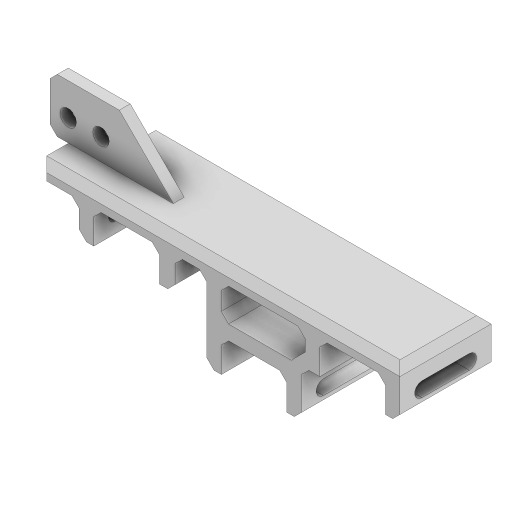
# Autodesk Inventor part: adapter_ver.1
Saved by Autodesk Inventor 2024 (Build 280153000, 153)
## iProperties
Created: 2023-11-09
Part Number: adapter_ver.1
Material: 一般
Document SubType Name: Modeling
Designer: moonshot
Density: 1 g/cm^3
Appearance: 既定
Author: moonshot
Autodesk Inventor part; units mm, degrees
ref_plane "YZ Plane" through (0, 0, 0) normal (1, 0, 0) x (0, 1, 0)
ref_plane "XZ Plane" through (0, 0, 0) normal (0, 1, 0) x (-1, 0, 0)
sketch "スケッチ1" plane through (0, 0, 0) normal (0, 0, 1) x (1, 0, 0)
  line L0 (94.5, 17.4383) -> (94.5, 4.4383)
  line L1 (67.5, 4.4383) -> (67.5, -8.5617)
  line L2 (0, -17.748) -> (0, 46.5561) projected
  line L3 (45.5, -8.5617) -> (45.5, 0.4383)
  line L4 (45.5, 0.4383) -> (63.5, 0.4383)
  line L5 (63.5, 0.4383) -> (63.5, -8.5617)
  line L6 (67.5, -8.5617) -> (63.5, -8.5617)
  line L7 (45.5, -8.5617) -> (41.5, -8.5617)
  line L8 (72.5, 4.4383) -> (72.5, 13.4383)
  line L9 (72.5, 13.4383) -> (90.5, 13.4383)
  line L10 (90.5, 13.4383) -> (90.5, 4.4383)
  line L11 (45.5, -8.5617) -> (55.5, -8.5617) construction
  line L12 (55.5, -8.5617) -> (55.5, 0.4383) construction
  line L13 (50.5, -8.5617) -> (50.5, 17.1682) construction
  line L14 (28.5, 4.4383) -> (28.5, 13.4383)
  line L15 (28.5, 13.4383) -> (10.5, 13.4383)
  line L16 (10.5, 13.4383) -> (10.5, 4.4383)
  line L17 (0, 17.4383) -> (0, 13.4383)
  line L18 (0, 17.4383) -> (94.5, 17.4383)
  line L19 (94.5, 4.4383) -> (90.5, 4.4383)
  line L20 (72.5, 4.4383) -> (67.5, 4.4383)
  line L21 (6.5, 4.4383) -> (10.5, 4.4383)
  line L22 (6.5, 4.4383) -> (6.5, 13.4383)
  line L23 (6.5, 13.4383) -> (0, 13.4383)
  line L24 (72.5, 4.4383) -> (82.5, 4.4383) construction
  line L25 (82.5, 4.4383) -> (82.5, 13.4383) construction
  line L26 (77.5, 4.4383) -> (77.5, 37.3698) construction
  line L27 (28.5, 4.4383) -> (18.5, 4.4383) construction
  line L28 (18.5, 4.4383) -> (18.5, 13.4383) construction
  line L29 (23.5, 4.4383) -> (23.5, 33.4166) construction
  line L30 (41.5, -8.5617) -> (41.5, 13.4383)
  line L31 (41.5, 13.4383) -> (32.8043, 13.4383)
  line L32 (32.8043, 13.4383) -> (32.8043, 4.4383)
  line L33 (32.8043, 4.4383) -> (28.5, 4.4383)
  line L34 (68.5, 13.4383) -> (45.5, 13.4383)
  line L35 (45.5, 13.4383) -> (45.5, 4.4383)
  line L36 (45.5, 4.4383) -> (64.698, 4.4383)
  line L37 (64.698, 4.4383) -> (68.5, 8.2403)
  line L38 (68.5, 8.2403) -> (68.5, 13.4383)
  point P0 (0, 0)
  point P1 (68.5, 10.8393)
  dimension "d5" = 4
  dimension "d10" = 18
  dimension "d14" = 18
  dimension "d16" = 10
  dimension "d19" = 9
  dimension "d23" = 4
  dimension "d40" = 4
  dimension "d41" = 9
  dimension "d42" = 10
  dimension "d43" = 10
  dimension "d44" = 50.5
  dimension "d74" = 4
  dimension "d89" = 4
  dimension "d90" = 135
  dimension "d91" = 4
  dimension "d92" = 4
  dimension "d93" = 4
  dimension "d94" = 4
  constraints: 76 end point, 24 perpendicular, 4 horizontal, 4 midpoint, 4 point on line, 4 symmetric about line, 3 vertical, 2 collinear
  measures "d5" distance of L3.start L7.end
  measures "d10" distance of L3.end L4.end
  measures "d14" distance of L8.end L9.end
  measures "d16" distance of L3.start L11.end
  measures "d19" distance of L3.start L3.end
  measures "d23" distance between parallel lines of L0 L10
  measures "d40" distance of L21.start L16.end
  measures "d41" distance of L8.start L8.end
  measures "d42" distance of L8.start L24.end
  measures "d43" distance of L14.start L27.end
  measures "d44" distance between parallel lines of L13 L2
  measures "d74" distance between parallel lines of L23 L18
  measures "d89" distance of L1.end L5.end
  measures "d90" angle of L37 L36
  measures "d91" distance from line of point (68.5, 10.839) L8
  measures "d92" distance between parallel lines of L18 L34
  measures "d93" distance between parallel lines of L30 L35
  measures "d94" distance between parallel lines of L4 L36
extrude "押し出し1" add sketch "スケッチ1" along normal mid plane 25
sketch "スケッチ2" plane through (67.5, -8.5617, 12.5) normal (1, 0, 0) x (0, 0, -1)
  line L0 (6, 3) -> (19, 3)
  arc A0 (19, 3) -> (19, 7) centre (19, 5) ccw
  line L1 (19, 7) -> (6, 7)
  arc A1 (6, 7) -> (6, 3) centre (6, 5) ccw
  line L2 (25, 0) -> (0, 0) projected
  line L3 (25, 13) -> (25, 0) projected
  line L4 (0, 0) -> (0, 13) projected
  point P0 (12.5, 8.5617)
  dimension "d24" = 4
  dimension "d25" = 3
  dimension "d26" = 6
  dimension "d27" = 6
  constraints: 4 end point, 4 point on circle, 4 tangent, 2 centre point, 1 horizontal, 1 parallel
  measures "d24" distance between parallel lines of L0 L1
  measures "d25" distance between parallel lines of L2 L0
  measures "d26" distance from line of L3 A0.centre
  measures "d27" distance from line of L4 A1.centre
extrude "押し出し2" cut sketch "スケッチ2" against normal up to surface (4 mm away)
chamfer "面取り1" distance 2 angle 45 1 edges at (63.5, 0.4383, 0)
sketch "スケッチ4" plane through (94.5, 4.4383, 12.5) normal (1, 0, 0) x (0, 0, -1)
  line L0 (6, 3) -> (19, 3)
  arc A0 (19, 3) -> (19, 7) centre (19, 5) ccw
  line L1 (19, 7) -> (6, 7)
  arc A1 (6, 7) -> (6, 3) centre (6, 5) ccw
  line L2 (25, 13) -> (25, 0) projected
  line L3 (0, 0) -> (0, 13) projected
  line L4 (25, 0) -> (0, 0) projected
  point P0 (12.5, -4.4383)
  dimension "d45" = 4
  dimension "d46" = 6
  dimension "d47" = 6
  dimension "d48" = 3
  constraints: 4 end point, 4 point on circle, 4 tangent, 2 centre point, 2 horizontal
  measures "d45" distance between parallel lines of L0 L1
  measures "d46" distance from line of L2 A0.centre
  measures "d47" distance from line of L3 A1.centre
  measures "d48" distance between parallel lines of L4 L0
extrude "押し出し3" cut sketch "スケッチ4" against normal up to surface (4 mm away)
sketch "スケッチ5" plane through (6.5, 4.4383, 12.5) normal (-1, 0, 0) x (0, 0, 1)
  line L0 (-19, 3) -> (-6, 3) projected
  line L1 (-19, 3) -> (-6, 3)
  arc A0 (-6, 3) -> (-6, 7) centre (-6, 5) ccw
  line L2 (-6, 7) -> (-19, 7) projected
  line L3 (-6, 7) -> (-19, 7)
  arc A1 (-19, 7) -> (-19, 3) centre (-19, 5) ccw
  point P0 (-12.5, -4.4383)
  point P1 (-6, 7)
  constraints: 4 end point, 4 point on circle, 4 tangent, 2 centre point, 2 equal length
extrude "押し出し4" cut sketch "スケッチ5" against normal up to surface (4 mm away)
chamfer "面取り4" distance 2 angle 45 3 edges at (90.5, 13.4383, 0) (10.5, 13.4383, 0) (6.5, 13.4383, 0)
ref_plane "作業平面1" through (0, 0, 1.5) normal (0, 0, 1) x (1, 0, 0)
sketch "スケッチ6" plane through (0, 0, 1.5) normal (0, 0, 1) x (1, 0, 0)
  line L0 (94.5, 17.4383) -> (0, 17.4383) projected
  line L1 (9.5, 17.4383) -> (-9.5, 17.4383)
  line L2 (-9.5, 17.4383) -> (-9.5, 32.2383)
  line L3 (-9.5, 32.2383) -> (9.5, 32.2383)
  line L4 (9.5, 32.2383) -> (9.5, 17.4383)
  line L5 (0, -5.8877) -> (0, 35.326) projected
  circle A0 centre (4.5, 23.4383) radius 2.25
  circle A1 centre (-4.5, 23.4383) radius 2.25
  point P0 (0, 0)
  dimension "d57" = 19
  dimension "d58" = 14.8
  dimension "d59" = 4.5
  dimension "d60" = 4.5
  dimension "d61" = 6
  constraints: 8 end point, 3 perpendicular, 2 centre point, 1 collinear, 1 point on line, 1 symmetric about line, 2 other
  measures "d57" distance of L2.end L3.end
  measures "d58" distance of L1.end L2.end
  measures "d59" diameter of A0
  measures "d60" distance from line of L5 A0.centre
  measures "d61" distance from line of L0 A0.centre
extrude "押し出し5" add sketch "スケッチ6" along normal blind 3
ref_plane "作業平面2" through (0, 0, 0.1) normal (0, 0, 1) x (1, 0, 0)
sketch "スケッチ7" plane through (0, 0, 0.1) normal (0, 0, 1) x (1, 0, 0)
  line L0 (-9.5, 17.4383) -> (0, 17.4383) projected
  line L1 (9.5, 17.4383) -> (0, 17.4383) projected
  line L2 (9.5, 17.4383) -> (9.5, 32.2383) projected
  line L3 (9.5, 32.2383) -> (-9.5, 32.2383) projected
  line L4 (-9.5, 32.2383) -> (-9.5, 17.4383) projected
  circle A0 centre (4.5, 23.4383) radius 2.25 projected
  circle A1 centre (-4.5, 23.4383) radius 2.25 projected
  line L5 (0, 13.4383) -> (4.5, 13.4383) projected
  line L6 (0, 17.4383) -> (0, 13.4383) projected
  line L7 (0, 13.4383) -> (0, 17.4383)
  line L8 (0, 17.4383) -> (-9.5, 17.4383)
  line L9 (-9.5, 17.4383) -> (0, 17.4383) projected
  line L10 (-4.4, 13.4383) -> (0, 13.4383)
  line L11 (-4.4, 13.4383) -> (-4.4, 17.4383)
  point P0 (0, 0)
  dimension "d70" = 4.4
  constraints: 8 end point, 2 collinear, 1 perpendicular, 1 point on line
  measures "d70" distance of L10.start L5.start
extrude "押し出し6" add sketch "スケッチ7" along normal up to surface (12.4 mm away) contours L0 L6 L10 L11
chamfer "面取り5" distance 14.8 angle 45 1 edges at (9.5, 17.4383, 3)
sketch "スケッチ8" plane through (0, 0, -12.5) normal (0, 0, -1) x (-1, 0, 0)
  line L0 (-4.5, 13.4383) -> (4.4, 13.4383) projected
  line L1 (-0.05, 13.4383) -> (-4.5, 13.4383)
  line L2 (-4.5, 13.4383) -> (0, 13.4383) projected
  line L3 (0, 13.4383) -> (0, 17.4383) projected
  line L4 (0, 17.4383) -> (-94.5, 17.4383) projected
  line L5 (-94.5, 17.4383) -> (-94.5, 4.4383) projected
  line L6 (-94.5, 4.4383) -> (-90.5, 4.4383) projected
  line L7 (-90.5, 4.4383) -> (-90.5, 11.4383) projected
  line L8 (-88.5, 13.4383) -> (-90.5, 11.4383) projected
  line L9 (-88.5, 13.4383) -> (-72.5, 13.4383) projected
  line L10 (-72.5, 13.4383) -> (-72.5, 4.4383) projected
  line L11 (-72.5, 4.4383) -> (-67.5, 4.4383) projected
  line L12 (-67.5, 4.4383) -> (-67.5, -8.5617) projected
  line L13 (-67.5, -8.5617) -> (-63.5, -8.5617) projected
  line L14 (-63.5, -8.5617) -> (-63.5, -1.5617) projected
  line L15 (-61.5, 0.4383) -> (-63.5, -1.5617) projected
  line L16 (-61.5, 0.4383) -> (-45.5, 0.4383) projected
  line L17 (-45.5, 0.4383) -> (-45.5, -8.5617) projected
  line L18 (-45.5, -8.5617) -> (-41.5, -8.5617) projected
  line L19 (-28.5, 4.4383) -> (-28.5, 13.4383) projected
  line L20 (-28.5, 13.4383) -> (-12.5, 13.4383) projected
  line L21 (-10.5, 11.4383) -> (-12.5, 13.4383) projected
  line L22 (-10.5, 11.4383) -> (-10.5, 4.4383) projected
  line L23 (-10.5, 4.4383) -> (-6.5, 4.4383) projected
  line L24 (-6.5, 4.4383) -> (-6.5, 11.4383) projected
  line L25 (-4.5, 13.4383) -> (-6.5, 11.4383) projected
  line L26 (-4.5, 13.4383) -> (-4.5, 17.4383)
  line L27 (0, 17.4383) -> (0, 13.4383)
  line L28 (0, 17.4383) -> (-4.5, 17.4383)
  line L29 (-41.5, -8.5617) -> (-41.5, 13.4383) projected
  line L30 (-41.5, 13.4383) -> (-32.8043, 13.4383) projected
  line L31 (-32.8043, 13.4383) -> (-32.8043, 4.4383) projected
  line L32 (-32.8043, 4.4383) -> (-28.5, 4.4383) projected
  point P0 (0, 0)
  point P1 (4.5, 13.4383)
  point P2 (-4.5, 13.4383)
  point P3 (0, 13.4383)
  dimension "d71" = 4.45
  constraints: 8 end point, 3 perpendicular, 3 point on line, 1 collinear, 1 midpoint
  measures "d71" distance of L1.start L0.start
extrude "押し出し7" cut sketch "スケッチ8" against normal blind 12.6 contours L26 L4 L3 L0
chamfer "面取り6" distance 2 angle 45 1 edges at (67.5, 4.4383, 0)
chamfer "面取り7" distance 2 angle 45 20 edges at (94.5, 17.4383, 0) (94.5, 4.4383, 0) (41.5, -8.5617, 0) (67.5, -8.5617, 0) (6.5, 4.4383, 0) (-9.5, 32.2383, 3) (-9.5, 17.4383, 3) (-4.4, 15.4383, 12.5) (4.5, 15.4383, -12.5) (28.5, 13.4383, 0) (45.5, 0.4383, 0) (72.5, 13.4383, 0) (45.05, 17.4383, 12.5) (49.5, 17.4383, -12.5) (68.5, 13.4383, 0) (45.5, 13.4383, 0) (45.5, 4.4383, 0) (32.8043, 4.4383, 0) (32.8043, 13.4383, 0) (41.5, 13.4383, 0)
